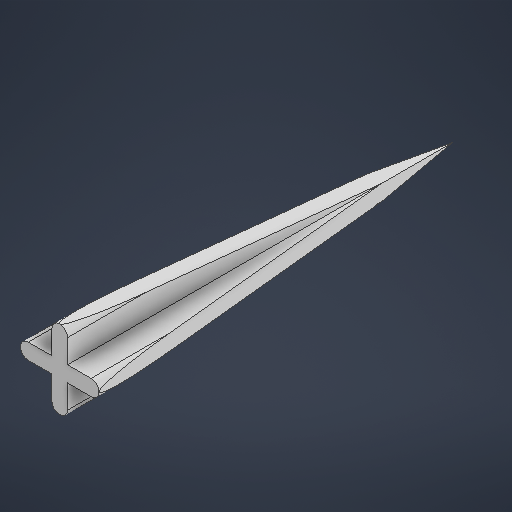
# Autodesk Inventor part: Prikker V1.1
Saved by Autodesk Inventor 2026.2 (Build 302298000, 298)
## iProperties
Created: 2026-04-21
Part Number: Prikker V1.1
Material: Generic
Document SubType Name: Modeling
Designer: thijs
Density: 1 g/cm^3
Appearance: Default
Author: thijs
Autodesk Inventor part; units mm, degrees
ref_plane "YZ Plane" through (0, 0, 0) normal (1, 0, 0) x (0, 1, 0)
ref_plane "XZ Plane" through (0, 0, 0) normal (0, 1, 0) x (-1, 0, 0)
ref_plane "XY Plane" through (0, 0, 0) normal (0, 0, 1) x (1, 0, 0)
sketch "Sketch1" plane through (0, 0, 0) normal (0, 0, 1) x (1, 0, 0)
  line L0 (0, 0) -> (0, -10)
  line L1 (0, 0) -> (10, 0)
  line L2 (0, 0) -> (0, 10)
  line L3 (0, 0) -> (-10, 0)
  line L4 (-10, 0) -> (-10, -2)
  line L5 (-10, -2) -> (0, -2)
  line L6 (-10, 0) -> (-10, 2)
  line L7 (-10, 2) -> (0, 2)
  line L8 (0, 10) -> (-2, 10)
  line L9 (-2, 10) -> (-2, 0)
  line L10 (0, 10) -> (2, 10)
  line L11 (2, 10) -> (2, 0)
  line L12 (0, 2) -> (10, 2)
  line L13 (10, 2) -> (10, 0)
  line L14 (10, -2) -> (0, -2)
  line L15 (10, -2) -> (10, 0)
  line L16 (2, 0) -> (2, -10)
  line L17 (0, -10) -> (2, -10)
  line L18 (0, -10) -> (-2, -10)
  line L19 (-2, -10) -> (-2, 0)
  line L20 (-10, 0) -> (-8, 0)
  line L21 (-8, 0) -> (-8, -2)
  line L22 (-8, 0) -> (-8, 2)
  arc A0 (-8, 2) -> (-10, 0) centre (-8, 0) ccw
  arc A1 (-10, 0) -> (-8, -2) centre (-8, 0) ccw
  line L23 (0, -10) -> (0, -8)
  line L24 (0, -8) -> (2, -8)
  line L25 (0, -8) -> (-2, -8)
  arc A2 (-2, -8) -> (0, -10) centre (0, -8) ccw
  arc A3 (0, -10) -> (2, -8) centre (0, -8) ccw
  line L26 (10, 0) -> (8, 0)
  line L27 (8, 0) -> (8, 2)
  line L28 (8, 0) -> (8, -2)
  arc A4 (8, -2) -> (10, 0) centre (8, 0) ccw
  arc A5 (10, 0) -> (8, 2) centre (8, 0) ccw
  line L29 (0, 10) -> (0, 8)
  line L30 (0, 8) -> (2, 8)
  line L31 (0, 8) -> (-2, 8)
  arc A6 (0, 10) -> (-2, 8) centre (0, 8) ccw
  arc A7 (2, 8) -> (0, 10) centre (0, 8) ccw
  point P0 (-2, -2)
  point P1 (2, -2)
  point P2 (2, 2)
  point P3 (-2, 2)
  dimension "d0" = 10
  dimension "d1" = 10
  dimension "d2" = 10
  dimension "d3" = 10
  dimension "d4" = 2
  dimension "d5" = 2
  dimension "d6" = 2
  dimension "d7" = 2
  dimension "d8" = 2
  dimension "d9" = 2
  dimension "d10" = 2
  dimension "d11" = 2
  dimension "d12" = 2
  dimension "d13" = 2
  dimension "d14" = 2
  dimension "d15" = 2
  dimension "d16" = 2
  dimension "d17" = 2
  dimension "d18" = 2
  constraints: 64 end point, 28 point on line, 16 point on circle, 12 perpendicular, 8 centre point, 3 vertical, 2 horizontal, 1 collinear, 1 concentric, 1 parallel
  measures "d0" distance of L0.start L0.end
  measures "d1" distance of L0.start L1.end
  measures "d2" distance of L0.start L2.end
  measures "d3" distance of L0.start L3.end
  measures "d4" distance of L3.end L4.end
  measures "d5" distance of L3.end L6.end
  measures "d6" distance of L2.end L8.end
  measures "d7" distance of L2.end L10.end
  measures "d8" distance of L3.end L20.end
  measures "d9" radius of A0
  measures "d10" radius of A1
  measures "d11" distance of L0.end L23.end
  measures "d12" radius of A2
  measures "d13" distance of L1.end L26.end
  measures "d14" radius of A4
  measures "d15" radius of A5
  measures "d16" distance of L2.end L29.end
  measures "d17" radius of A6
  measures "d18" radius of A7
extrude "Extrusion1" add sketch "Sketch1" along normal blind 100 contours L1 L16 L14 L0 | L2 L12 L11 L1 | L3 L9 L7 L2 | L0 L5 L19 L3 | L14 L16 L24 L0 | L0 L25 L19 L5 | L11 L12 L27 L1 | L1 L28 L14 L16 | L7 L9 L31 L2 | L2 L30 L11 L12 | L19 L5 L21 L3 | L3 L22 L7 L9 | L24 A3 L0 | L0 A2 L25 | L27 A5 L1 | L1 A4 L28 | L31 A6 L2 | L2 A7 L30 | L21 A1 L3 | L3 A0 L22
sketch "Sketch2" plane through (0, 0, 0) normal (0, 1, 0) x (-1, 0, 0)
  line L0 (2, 100) -> (-2, 100) projected
  line L1 (10, 0) -> (10, 100) projected
  line L2 (2, 100) -> (2, 0)
  line L3 (10, 100) -> (2, 100)
  line L4 (-2, 100) -> (-2, 0)
  line L5 (-8, 100) -> (-10, 100) projected
  line L6 (-10, 100) -> (-2, 100)
  line L7 (10, 0) -> (10, 100)
  line L8 (-2, 0) -> (-10, 0)
  line L9 (-10, 0) -> (-10, 100)
  line L10 (10, 0) -> (0, 0)
  line L11 (0, 0) -> (10, 100)
  line L12 (0, 0) -> (-10, 100)
  line L13 (-10, 0) -> (0, 0)
  line L14 (0, 0) -> (-10, 100)
  constraints: 24 end point, 3 collinear, 2 horizontal, 1 perpendicular, 1 vertical
extrude "Extrusion2" cut sketch "Sketch2" along normal mid plane 20 contours L11 L1 L10 L2 | L2 L10 L11 | L12 L13 L4 | L4 L8 L9 L12
sketch "Sketch3" plane through (0, 0, 0) normal (1, 0, 0) x (0, 1, 0)
  line L0 (0, 100) -> (-2, 100) projected
  line L1 (0, 0) -> (0, 100)
  line L2 (0, 100) -> (10, 100)
  line L3 (10, 0) -> (10, 100) projected
  line L4 (10, 100) -> (10, 0)
  line L5 (-10, 0) -> (10, 0) projected
  line L6 (0, 0) -> (10, 0)
  line L7 (10, 0) -> (0, 0)
  line L8 (10, 100) -> (0, 0)
  line L9 (0, 0) -> (-10, 0)
  line L10 (-10, 0) -> (-10, 100)
  line L11 (-10, 100) -> (0, 100)
  line L12 (-10, 100) -> (0, 0)
  constraints: 20 end point, 3 perpendicular, 3 point on line, 2 collinear, 1 horizontal, 1 vertical
extrude "Extrusion3" cut sketch "Sketch3" along normal mid plane 20 contours L8 L3 L5 | L5 L10 L12
sketch "Sketch4" plane through (0, 0, 100) normal (0, 0, 1) x (1, 0, 0)
  line L0 (-8, -2) -> (-2, -2) projected
  line L1 (-2, -2) -> (-8, -2)
  line L2 (-2, -2) -> (-2, -7.923)
  line L3 (2, -8) -> (2, -2) projected
  line L4 (2, -2) -> (2, -8)
  arc A0 (8, -2) -> (10, 0) centre (8, 0) ccw projected
  line L5 (2, -2) -> (8, -2)
  line L6 (2, 2) -> (2, 8) projected
  line L7 (8, 2) -> (2, 2) projected
  line L8 (2, 2) -> (8, 2)
  line L9 (2, 2) -> (2, 8)
  line L10 (-2, 8) -> (-2, 2) projected
  line L11 (-2, 2) -> (-2, 8)
  arc A1 (-8, 2) -> (-10, 0) centre (-8, 0) ccw projected
  line L12 (-2, 2) -> (-8, 2)
  arc A2 (-8, 2) -> (-8, -2) centre (-8, 0) ccw
  arc A3 (-2, -8) -> (0, -10) centre (0, -8) ccw projected
  arc A4 (-2, -8) -> (2, -8) centre (0, -8) ccw
  arc A5 (8, -2) -> (8, 2) centre (8, 0) ccw
  arc A6 (2, 8) -> (-2, 8) centre (0, 8) ccw
  constraints: 16 end point, 11 point on circle, 9 tangent, 4 centre point, 3 collinear, 3 horizontal, 1 perpendicular, 1 vertical
body "Solid1"
